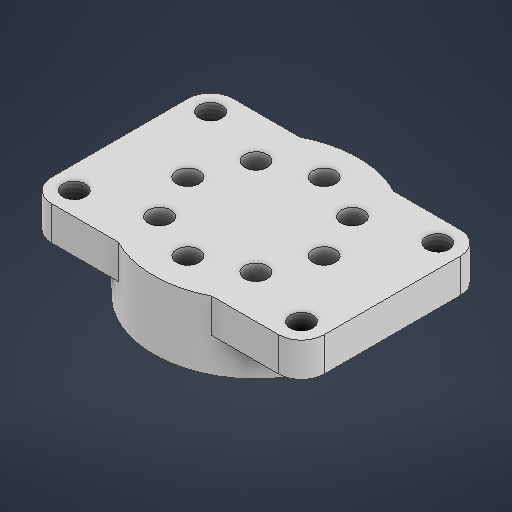
# Autodesk Inventor part: ArmBearingClampingPlate1
Saved by Autodesk Inventor 2025 (Build 290162000, 162)
## iProperties
Created: 2024-05-20
Part Number: ArmBearingClampingPlate1
Material: Generic
Document SubType Name: Modeling
Designer: avsar
Density: 1 g/cm^3
Appearance: Default
Author: avsar
Autodesk Inventor part; units mm, degrees
ref_plane "YZ Plane" through (0, 0, 0) normal (1, 0, 0) x (0, 1, 0)
ref_plane "XZ Plane" through (0, 0, 0) normal (0, 1, 0) x (-1, 0, 0)
ref_plane "XY Plane" through (0, 0, 0) normal (0, 0, 1) x (1, 0, 0)
sketch "Sketch1" plane through (0, 0, 0) normal (0, 1, 0) x (-1, 0, 0)
  circle A0 centre (0, 0) radius 18
  dimension "d0" = 36
  constraints: 1 centre point, 1 coincident
  measures "d0" diameter of A0
extrude "Extrusion1" add sketch "Sketch1" along normal blind 6
sketch "Sketch2" plane through (0, 6, 0) normal (0, 1, 0) x (1, 0, 0)
  circle A0 centre (0, 12) radius 2
  circle A1 centre (-8.4853, 8.4853) radius 2
  circle A2 centre (-12, 0) radius 2
  circle A3 centre (-8.4853, -8.4853) radius 2
  circle A4 centre (0, -12) radius 2
  circle A5 centre (8.4853, -8.4853) radius 2
  circle A6 centre (12, 0) radius 2
  circle A7 centre (8.4853, 8.4853) radius 2
  point P0 (0, 0)
  dimension "d3" = 4
  dimension "d4" = 12
  dimension "d7" = 360
  constraints: 8 centre point, 1 vertical alignment, 17 other
  measures "d3" diameter of A0
  measures "d4" distance of point (0, 0) A0.centre
extrude "Extrusion2" cut sketch "Sketch2" against normal through all
sketch "Sketch3" plane through (0, 6, 0) normal (0, 1, 0) x (1, 0, 0)
  line L0 (-24, -16) -> (24, -16)
  line L1 (24, -16) -> (24, 16)
  line L2 (24, 16) -> (-24, 16)
  line L3 (-24, 16) -> (-24, -16)
  line L4 (-24, -16) -> (24, 16) construction
  line L5 (24, -16) -> (-24, 16) construction
  circle A0 centre (20, -12) radius 2
  line L6 (0, 0) -> (0, 16) construction
  line L7 (0, 0) -> (-24, 0) construction
  circle A1 centre (20, 12) radius 2
  circle A2 centre (-20, -12) radius 2
  circle A3 centre (-20, 12) radius 2
  circle A4 centre (0, 0) radius 18 projected
  circle A5 centre (0, -12) radius 2 projected
  circle A6 centre (12, 0) radius 2 projected
  circle A7 centre (-8.4853, 8.4853) radius 2 projected
  circle A8 centre (-8.4853, -8.4853) radius 2 projected
  circle A9 centre (-12, 0) radius 2 projected
  circle A10 centre (0, 12) radius 2 projected
  circle A11 centre (8.4853, -8.4853) radius 2 projected
  circle A12 centre (8.4853, 8.4853) radius 2 projected
  circle A13 centre (0, 0) radius 18 projected
  point P0 (-8.2462, 16)
  point P1 (-8.2462, -16)
  point P2 (8.2462, -16)
  point P3 (8.2462, 16)
  dimension "d11" = 48
  dimension "d12" = 32
  dimension "d13" = 4
  dimension "d14" = 20
  dimension "d15" = 12
  constraints: 16 end point, 4 centre point, 4 midpoint, 3 symmetric about line, 2 parallel, 1 horizontal, 1 perpendicular, 3 other
  measures "d11" distance of L2.end L1.end
  measures "d12" distance of L1.end L0.end
  measures "d13" diameter of A0
  measures "d14" horizontal distance of L6.start A0.centre
  measures "d15" vertical distance of L6.start A0.centre
extrude "Extrusion3" add sketch "Sketch3" along normal blind 6
fillet "Fillet1" radius 4 4 edges at (24, 9, -16) (24, 9, 16) (-24, 9, -16) (-24, 9, 16)
thread "Thread1" size "M4x0.7" class "6H" standard "ANSI Metric M Profile" full length
thread "Thread2" size "M4x0.7" class "6H" standard "ANSI Metric M Profile" full length
thread "Thread3" size "M4x0.7" class "6H" standard "ANSI Metric M Profile" full length
thread "Thread4" size "M4x0.7" class "6H" standard "ANSI Metric M Profile" full length
body "Solid1"
